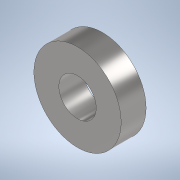
# Autodesk Inventor part: Ball Bearing-1
Saved by Autodesk Inventor 2021.1 (Build 251245010, 245A)
## iProperties
Created: 2025-09-16
Part Number: Ball Bearing-1
Material: Steel, Alloy
Document SubType Name: Modeling
Designer: SD
Density: 7.73 g/cm^3
Appearance: Semi-Polished
Mass: 0.48569 g
Surface Area: 1.25664 cm^2
Volume: 0.0628319 cm^3
Project: Automatic Tea Steeping mechanism
BOM-Mass: 0.00049
BOM-Area: 0.000
Author: SD
Title: Ball Bearing-1
Autodesk Inventor part; units mm, degrees
ref_plane "YZ Plane" through (0, 0, 0) normal (1, 0, 0) x (0, 1, 0)
ref_plane "XZ Plane" through (0, 0, 0) normal (0, 1, 0) x (-1, 0, 0)
ref_plane "XY Plane" through (0, 0, 0) normal (0, 0, 1) x (1, 0, 0)
sketch "Sketch1" plane through (0, 0, 0) normal (0, 0, 1) x (1, 0, 0)
  circle A0 centre (0, 0) radius 3.5
  circle A1 centre (0, 0) radius 1.5
  dimension "d0" = 7
  dimension "d1" = 3
  constraints: 2 centre point, 2 coincident
  measures "d0" diameter of A0
  measures "d1" diameter of A1
extrude "Extrusion1" add sketch "Sketch1" along normal mid plane 2
body "Solid1"
